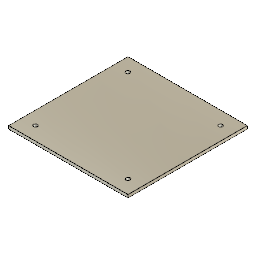
bed v2 (Autodesk Fusion 360 design; units mm, degrees)
Autodesk Fusion 360 part; units mm, degrees
sketch "Sketch1" plane through (0, 0, 0) normal (0, 0, 1) x (1, 0, 0)
  line L0 (155, -155) -> (-155, -155)
  line L1 (-155, -155) -> (-155, 155)
  line L2 (-155, 155) -> (155, 155)
  line L3 (155, 155) -> (155, -155)
  line L4 (155, -155) -> (-155, 155) construction
  line L5 (-155, -155) -> (155, 155) construction
  line L6 (120, -120) -> (-120, -120) construction
  line L7 (-120, -120) -> (-120, 120) construction
  line L8 (-120, 120) -> (120, 120) construction
  line L9 (120, 120) -> (120, -120) construction
  line L10 (120, -120) -> (-120, 120) construction
  line L11 (-120, -120) -> (120, 120) construction
  circle A0 centre (120, 120) radius 5
  circle A1 centre (120, -120) radius 5
  circle A2 centre (-120, -120) radius 5
  circle A3 centre (-120, 120) radius 5
  circle A4 centre (0, 0) radius 150
  dimension "d1" = 310
  dimension "d2" = 310
  dimension "d3" = 240
  dimension "d4" = 240
  dimension "d5" = 10
  dimension "d6" = 10
  dimension "d7" = 10
  dimension "d8" = 10
  dimension "d9" = 300
  constraint perpendicular L0 L1
  constraint parallel L0 L2
  constraint parallel L1 L3
  constraint horizontal L0
  constraint coincident L4 A4.centre
  constraint coincident L5 A4.centre
  constraint coincident A4.centre origin
  constraint perpendicular L6 L7
  constraint parallel L6 L8
  constraint parallel L7 L9
  constraint horizontal L6
  constraint coincident L10 A4.centre
  constraint coincident L11 A4.centre
  constraint coincident L8.end L9.start
  constraint coincident L6.start L9.end
  constraint coincident L6.end L7.start
  constraint coincident L7.end L8.start
  measures "d1" distance of L0.end L1.end
  measures "d2" distance of L1.end L2.end
  measures "d3" distance of L7.end L8.end
  measures "d4" distance of L6.end L7.end
  measures "d5" diameter of A0
  measures "d6" diameter of A1
  measures "d7" diameter of A2
  measures "d8" diameter of A3
  measures "d9" diameter of A4
extrude "Extrude1" add sketch "Sketch1" along normal blind 8 contours L0 L1 L2 L3 | A4 makes body 1
extrude "Extrude2" add sketch "Sketch1" against normal blind 3 separate body contours A4 makes body 2
equation "d6 = d5"
equation "d7 = d5"
equation "d8 = d5"
